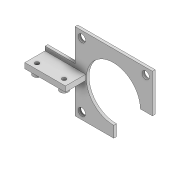
# Autodesk Inventor part: stop_rotador_2
Saved by Autodesk Inventor 2022 (Build 260153000, 153)
## iProperties
Created: 2023-03-25
Part Number: stop_rotador_2
Material: Generic
Document SubType Name: Modeling
Designer: ferna
Density: 1 g/cm^3
Appearance: Default
Author: ferna
Autodesk Inventor part; units mm, degrees
ref_plane "YZ Plane" through (0, 0, 0) normal (1, 0, 0) x (0, 1, 0)
ref_plane "XZ Plane" through (0, 0, 0) normal (0, 1, 0) x (-1, 0, 0)
ref_plane "XY Plane" through (0, 0, 0) normal (0, 0, 1) x (1, 0, 0)
sketch "Sketch1" plane through (0, 0, 0) normal (0, 0, 1) x (1, 0, 0)
  line L0 (30.9017, 120.8967) -> (30.9017, 145.8967)
  line L1 (30.9017, 145.8967) -> (-30.2983, 145.8967)
  line L2 (-30.2983, 145.8967) -> (-30.2983, 120.8967)
  line L3 (-30.2983, 120.8967) -> (-33.2983, 120.8967)
  line L4 (-33.2983, 120.8967) -> (-33.2983, 89.6967)
  line L5 (-33.2983, 89.6967) -> (-25.2983, 81.6967)
  line L6 (-25.2983, 81.6967) -> (25.9017, 81.6967)
  line L7 (25.9017, 81.6967) -> (33.9017, 89.6967)
  line L8 (33.9017, 89.6967) -> (33.9017, 120.8967)
  line L9 (33.9017, 120.8967) -> (30.9017, 120.8967)
  circle A0 centre (0, 115) radius 20
  circle A1 centre (-23.2983, 138.8967) radius 2.75
  circle A2 centre (23.9017, 91.6967) radius 2.75
  circle A3 centre (23.9017, 138.8967) radius 2.75
  circle A4 centre (-23.2983, 91.6967) radius 2.75
  line L10 (-30.2983, 145.8967) -> (-30.2983, 143.8967)
  line L11 (-30.2983, 143.8967) -> (-28.2983, 143.8967)
  line L12 (-28.2983, 143.8967) -> (28.9017, 143.8967)
  line L13 (28.9017, 143.8967) -> (28.9017, 86.6967)
  line L14 (28.9017, 86.6967) -> (-28.2983, 86.6967)
  line L15 (-28.2983, 86.6967) -> (-28.2983, 143.8967)
  line L16 (0.3017, 86.6967) -> (0.3017, 95.0023)
  line L17 (19.9978, 115.2967) -> (28.9017, 115.2967)
  point P0 (0, 0)
  dimension "d0" = 2
  dimension "d1" = 57.2
  constraints: 36 end point, 5 centre point, 3 perpendicular, 2 midpoint, 2 parallel, 2 point on circle, 2 point on line
  measures "d0" distance of L1.end L10.end
  measures "d1" distance of L11.end L12.end
extrude "Extrusion1" add sketch "Sketch1" along normal blind 2 contours L12 L13 L17 A0 L16 L14 L15
sketch "Sketch6" plane through (0, 0, 2) normal (0, 0, 1) x (1, 0, 0)
  line L0 (-36.1687, 110.2967) -> (-20.428, 110.2967)
  line L1 (-20.428, 110.2967) -> (-20.428, 120.2967)
  line L2 (-20.428, 120.2967) -> (-36.1687, 120.2967)
  line L3 (-36.1687, 120.2967) -> (-36.1687, 110.2967)
  line L4 (-28.2983, 143.8967) -> (-28.2983, 86.6967) projected
  line L5 (-36.1687, 110.2967) -> (-20.428, 120.2967) construction
  line L6 (-20.428, 110.2967) -> (-36.1687, 120.2967) construction
  line L7 (-20.428, 120.2967) -> (-50.428, 120.2967)
  line L8 (-50.428, 120.2967) -> (-50.428, 110.2967)
  line L9 (-50.428, 110.2967) -> (-20.428, 110.2967)
  point P0 (0, 0)
  point P1 (-28.2983, 115.2967)
  dimension "d14" = 10
  dimension "d17" = 30
  constraints: 18 end point, 3 midpoint, 2 parallel, 2 perpendicular, 1 collinear, 1 horizontal, 1 point on line
  measures "d14" distance of L1.end L0.end
  measures "d17" distance of L1.end L7.end
extrude "Extrusion5" add sketch "Sketch6" against normal blind 2
sketch "Sketch7" plane through (0, 0, 2) normal (0, 0, 1) x (1, 0, 0)
  line L0 (-50.428, 110.2967) -> (-50.428, 120.2967) projected
  line L1 (-50.428, 115.2967) -> (-50.428, 117.2967)
  line L2 (-50.428, 117.2967) -> (-20.428, 117.2967)
  line L3 (-20.428, 117.2967) -> (-20.428, 113.2967)
  line L4 (-20.428, 113.2967) -> (-50.428, 113.2967)
  line L5 (-50.428, 113.2967) -> (-50.428, 115.2967)
  point P0 (0, 0)
  dimension "d18" = 2
  dimension "d19" = 30
  dimension "d20" = 4
  constraints: 10 end point, 4 perpendicular, 2 point on line, 1 midpoint
  measures "d18" distance of L1.start L1.end
  measures "d19" distance of L1.end L2.end
  measures "d20" distance of L2.end L3.end
extrude "Extrusion6" add sketch "Sketch7" along normal blind 15
sketch "Sketch8" plane through (-50.428, 113.2967, 2) normal (0, -1, 0) x (1, 0, 0)
  circle A0 centre (25, 11) radius 3
  circle A1 centre (5, 11) radius 3
  line L0 (30, 15) -> (30, 7)
  line L1 (30, 15) -> (0, 15)
  line L2 (0, 7) -> (0, 15)
  line L3 (30, 7) -> (0, 7)
  circle A2 centre (25, 11) radius 3
  circle A3 centre (25, 11) radius 1.5
  circle A4 centre (5, 11) radius 1.5
  circle A5 centre (5, 11) radius 3
  circle A6 centre (5, 11) radius 1.5
  point P0 (50.428, -2)
  constraints: 8 end point, 7 centre point
extrude "Extrusion7" add sketch "Sketch8" along normal blind 3 contours A0 | A1
sketch "Sketch9" plane through (-50.428, 113.2967, 2) normal (0, -1, 0) x (1, 0, 0)
  circle A0 centre (25, 11) radius 1.5 projected
  circle A1 centre (5, 11) radius 1.5 projected
  point P0 (50.428, -2)
extrude "Extrusion8" cut sketch "Sketch9" against normal through all
body "Solid1"
